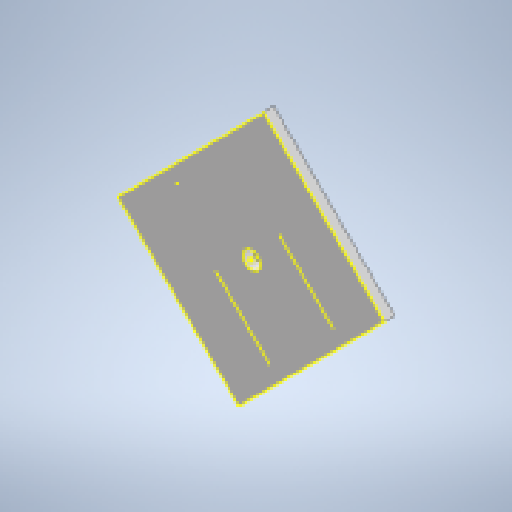
# Autodesk Inventor part: _body_2_
Saved by Autodesk Inventor 2024.3 (Build 283343000, 343)
## iProperties
Created: 2024-09-06
Part Number: _body_2_
Material: 일반
Document SubType Name: Modeling
Designer: gretc
Density: 1 g/cm^3
Appearance: 기본값
Author: gretc
Autodesk Inventor part; units mm, degrees
ref_plane "YZ Plane" through (0, 0, 0) normal (1, 0, 0) x (0, 1, 0)
ref_plane "XZ Plane" through (0, 0, 0) normal (0, 1, 0) x (-1, 0, 0)
ref_plane "XY Plane" through (0, 0, 0) normal (0, 0, 1) x (1, 0, 0)
ref_plane "작업 평면1" through (0, 0, 0) normal (0, 0, 1) x (1, 0, 0)
sketch "스케치1" plane through (0, 0, 0) normal (0, 0, 1) x (1, 0, 0)
  line L0 (-7.4991, -77.3538) -> (77.3538, 7.4991) projected
  circle A0 centre (0, 0) radius 7.5 projected
  circle A1 centre (-16.0513, 40.5172) radius 1.35 projected
  circle A2 centre (-24.9609, 0.495) radius 1.35 projected
  circle A3 centre (-40.5172, 16.0513) radius 1.35 projected
  circle A4 centre (-0.495, 24.9609) radius 1.35 projected
  circle A5 centre (-24.2538, 39.8101) radius 1.35 projected
  circle A6 centre (-9.4045, -15.0614) radius 1.35 projected
  circle A7 centre (-39.8101, 24.2538) radius 1.35 projected
  circle A8 centre (15.0614, 9.4045) radius 1.35 projected
  line L1 (6.6431, 78.2097) -> (-78.2097, -6.6431) projected
  line L2 (-78.2097, -6.6431) -> (-7.4991, -77.3538) projected
  line L3 (-7.4991, -77.3538) -> (77.3538, 7.4991) projected
  line L4 (77.3538, 7.4991) -> (6.6431, 78.2097) projected
  circle A9 centre (46.7785, -2.3722) radius 1.35 projected
  circle A10 centre (53.2838, 4.1332) radius 1.35 projected
  circle A11 centre (3.2773, 54.1398) radius 1.35 projected
  circle A12 centre (-3.6698, 47.1928) radius 1.35 projected
  circle A13 centre (-47.1928, 3.6698) radius 1.35 projected
  circle A14 centre (-54.1398, -3.2773) radius 1.35 projected
  circle A15 centre (2.3722, -46.7785) radius 1.35 projected
  circle A16 centre (-4.1332, -53.2838) radius 1.35 projected
  line L5 (7.0711, 77.7817) -> (-77.7817, -7.0711)
  line L6 (-77.7817, -7.0711) -> (-7.0711, -77.7817)
  line L7 (-7.0711, -77.7817) -> (77.7817, 7.0711)
  line L8 (77.7817, 7.0711) -> (7.0711, 77.7817)
  line L9 (7.0711, 77.7817) -> (-7.0711, -77.7817) construction
  line L10 (-77.7817, -7.0711) -> (77.7817, 7.0711) construction
  circle A17 centre (0, 0) radius 5 projected
  point P0 (0, 0)
  point P1 (-77.7817, -7.0711)
  dimension "d0" = 100
  constraints: 12 end point, 2 midpoint, 2 parallel, 2 perpendicular
  measures "d0" distance of L6.end L5.end
extrude "돌출1" add sketch "스케치1" along normal blind 6 contours L2 L5 L4 L0 | A0 | A1 | A2 | A3 | A4 | A5 | A6 | A7 | A8 | A9 | A10 | A11 | A12 | A13 | A14 | A15 | A16
sketch "스케치2" plane through (-7.4991, -77.3538, 6) normal (-0.7071068, -0.7071068, 0) x (-0.7071068, 0.7071068, 0)
  line L0 (99.3947, 6) -> (0, 6) projected
  line L1 (0, 6) -> (0, 0) projected
  line L2 (99.3947, 0) -> (0, 0) projected
  line L3 (99.3947, 6) -> (99.3947, 0) projected
  point P0 (49.3947, 6)
sketch "스케치3" plane through (7.0711, 77.7817, 0) normal (0.7071068, 0.7071068, 0) x (-0.7071068, 0.7071068, 0)
  line L0 (-99.3947, 0) -> (0, 0) projected
  line L1 (0, 0) -> (0, 6) projected
  line L2 (-99.3947, 6) -> (0, 6) projected
  line L3 (-99.3947, 0) -> (-99.3947, 6) projected
  point P0 (-50, 0)
extrude "돌출2" add sketch "스케치3" along normal blind 6
